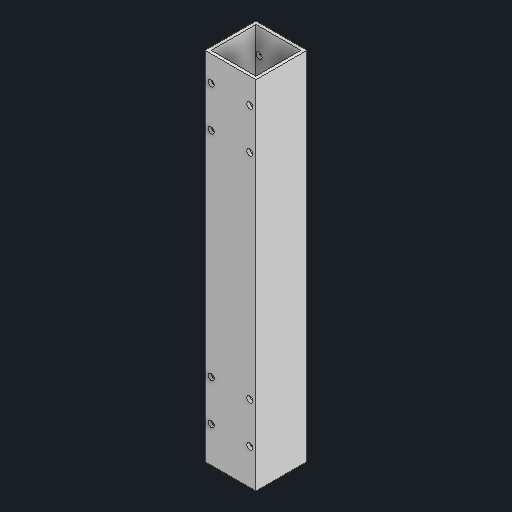
# Autodesk Inventor part: femur_profile
Saved by Autodesk Inventor 2026 (Build 300175000, 175)
## iProperties
Created: 2026-04-24
Part Number: femur_profile
Material: Типовые
Document SubType Name: Modeling
Designer: user
Density: 1 g/cm^3
Appearance: По умолчанию
Mass: 195.997 g
Surface Area: 1327.13 cm^2
Volume: 195.997 cm^3
Author: user
Autodesk Inventor part; units mm, degrees
ref_plane "YZ Plane" through (0, 0, 0) normal (1, 0, 0) x (0, 1, 0)
ref_plane "XZ Plane" through (0, 0, 0) normal (0, 1, 0) x (-1, 0, 0)
ref_plane "XY Plane" through (0, 0, 0) normal (0, 0, 1) x (1, 0, 0)
sketch "Эскиз1" plane through (0, 0, 0) normal (0, 1, 0) x (-1, 0, 0)
  line L0 (0, 0) -> (50, 0)
  line L1 (50, 0) -> (50, -50)
  line L2 (50, -50) -> (0, -50)
  line L3 (0, -50) -> (0, 0)
  line L4 (3, -47) -> (47, -47)
  line L5 (47, -47) -> (47, -3)
  line L6 (47, -3) -> (3, -3)
  line L7 (3, -3) -> (3, -47)
  dimension "d0" = 50
  dimension "d1" = 50
  dimension "d2" = 3
  constraints: 16 end point, 4 parallel, 2 perpendicular, 1 horizontal, 3 other
  measures "d0" distance of L1.end L2.end
  measures "d1" distance of L2.end L0.start
  measures "d2" distance between parallel lines of L3 L7
extrude "Выдавливание1" add sketch "Эскиз1" along normal blind 350
sketch "Эскиз2" plane through (-50, 0, 0) normal (0, 0, 1) x (1, 0, 0)
  line L0 (0, 0) -> (50, 0) projected
  line L1 (50, 0) -> (50, 350) projected
  line L2 (0, 350) -> (50, 350) projected
  line L3 (0, 0) -> (0, 350) projected
  circle A0 centre (43.95, 325) radius 3.05
  circle A1 centre (43.95, 285) radius 3.05
  circle A2 centre (6.05, 325) radius 3.05
  circle A3 centre (6.05, 285) radius 3.05
  line L4 (3, 0) -> (47, 0) projected
  line L5 (47, 0) -> (47, 350) projected
  line L6 (3, 350) -> (47, 350) projected
  line L7 (3, 0) -> (3, 350) projected
  circle A4 centre (6.05, 35) radius 3.05
  circle A5 centre (43.95, 35) radius 3.05
  circle A6 centre (43.95, 75) radius 3.05
  circle A7 centre (6.05, 75) radius 3.05
  dimension "d5" = 6.1
  dimension "d8" = 40
  dimension "d11" = 37.9
  dimension "d14" = 25
  dimension "d15" = 6.05
  dimension "d18" = 6.1
  dimension "d19" = 35
  dimension "d22" = 40
  constraints: 8 centre point, 2 tangent, 2 vertical, 1 equal radius, 1 horizontal, 1 horizontal alignment, 10 other
  measures "d5" diameter of A0
  measures "d8" distance of A0.centre A1.centre
  measures "d11" distance of A0.centre A2.centre
  measures "d14" distance from line of L2 A2.centre
  measures "d15" distance from line of L1 A0.centre
  measures "d18" diameter of A5
  measures "d19" distance from line of L4 A4.centre
  measures "d22" distance of A5.centre A6.centre
extrude "Выдавливание2" cut sketch "Эскиз2" against normal through all contours A5 | A6 | A1 | A0 | A2 | A3 | A7 | A4
equation "\"d0\" = width_profile_femur"
equation "\"d1\" = hight_profile_femur"
equation "\"d2\" = thickness_profile_femur"
equation "\"d3\" = length_profile_femur"
equation "\"d5\" = d_main_screw_holes"
equation "\"d11\" = -2 * thickness_profile_femur + hight_profile_femur - d_main_screw_holes"
equation "\"d15\" = 0.5 * d_main_screw_holes + thickness_profile_femur"
equation "\"d18\" = d_main_screw_holes"
equation "\"tolerance_plazma\" = 0.1"
equation "\"thickness_steel\" = 3"
equation "\"d_main_screw_holes\" = 6.1"
equation "\"thickness_profile_tibea\" = 4"
equation "\"thickness_profile_femur\" = 3"
equation "\"width_profile_femur\" = 50"
equation "\"width_shaft_shift\" = 35"
equation "\"length_profile_femur\" = 350"
equation "\"hight_profile_femur\" = 50"
equation "\"width_flattened_surface\" = 12"
